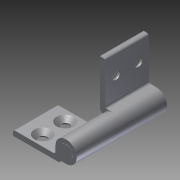
# Autodesk Inventor part: MayTec 1.62.842032085_Alu hinges, heavy, type 20 PG 40 (90)
Saved by Autodesk Inventor 2011 SP1 (Build 150282100, 282)
## iProperties
Created: 2012-12-11
Part Number: MayTec 1.62.842032085_Alu hinges, heavy, type 20 PG 40 (90)
Catalog Web Link: www.cadenas.de
Description: Alu hinges, heavy-Alu hinges, heavy
Vendor: MAYTEC
Document SubType Name: Modeling
Designer: PARTuser1
Manufacturer: MAYTEC
Density: 1 g/cm^3
Category: PARTsolutions
Company: MAYTEC
Title: MayTec 1.62.842032085_Alu hinges, heavy, type 20 PG 40 (90)
Author: Cadenas PARTsolutions
Comments: Alu hinges, heavy
PSOL_IDENT_0: {\\10.0.0.242\data_v9\23d-libs\maytec\maytec_3d\anbauzubehoer\scharniere\alu_scharniere\alu_scharnie
PSOL_IDENT_1: r_schwer.prj},278 {VTYP=3D},{NB=MayTec 1.62.842032085_Alu hinges, heavy, type 20 PG 40 (90)},{LINA=M
PSOL_IDENT_2: ayTec 1.62.842032085_Alu hinges, heavy, type 20 PG 40 (90)},{NN=Alu hinges, heavy},{DATE=14.09.2010
PSOL_IDENT_3: 08:32:09},{GEOMDATE=27.07.2010 11:58:00},{VERSION=},{LINEID=250},{LINESUBID=-1},{WBVAR=WINKEL}  {NB=
PSOL_IDENT_4: MayTec 1.62.842032085_Alu hinges, heavy, type 20 PG 40 (90)},{LINA=MayTec 1.62.842032085_Alu hinges,
PSOL_IDENT_5: heavy, type 20 PG 40 (90)},{KT=DUMMY},{PARTNR=1.62.842032085},{DESCRIPTION=Alu-Scharnier-Schwer Typ
PSOL_IDENT_6: 20 PG 40},{TYP=20.0},{AUSFHRUNG=Stahl},{H=128.75},{A=32.0},{T=20.0},{T2=86.00},{VAR=1.0},{XTRANS=Al
PSOL_IDENT_7: u hinges, heavy, type 20 PG 40},{B=100},{WINKEL=90}
CNS_NT: Alu hinges, heavy
CNS_NB: MayTec 1.62.842032085_Alu hinges, heavy, type 20 PG 40 (90)
CNS_NBSYN: MayTec $PARTNR._$XTRANS. ($WINKEL.)
CNS_LINA: MayTec 1.62.842032085_Alu hinges, heavy, type 20 PG 40 (90)
CNS_PARTNR: 1.62.842032085
CNS_DESCRIPTION: Alu hinges, heavy, type 20 PG 40
CNS_TYP: 20.0
CNS_AUSFHRUNG: Steel
CNS_H: 128.75
CNS_A: 32.0
CNS_T: 20.0
CNS_T2: 86.00
CNS_VAR: 1.0
CNS_XTRANS: Alu hinges, heavy, type 20 PG 40
CNS_B: 100
CNS_WINKEL: 90
SUPPLIER: MAYTEC
ARTICLENO: MayTec 1.62.842032085_Alu hinges, heavy, type 20 PG 40 (90)
BOMINFO: MayTec 1.62.842032085_Alu hinges, heavy, type 20 PG 40 (90)
CREATOR: CADENAS GmbH
Autodesk Inventor part; units mm, degrees
sketch "Skizze_34" plane through (0, 0, 0) normal (0, 1, 0) x (1, 0, 0)
  circle A0 centre (0, 12) radius 10
  constraints: 1 centre point
extrude "Extrusion1" add sketch "Skizze_34" along normal mid plane 2.5
sketch "Skizze_35" plane through (0, 0, 0) normal (0, 1, 0) x (1, 0, 0)
  circle A0 centre (0, 12) radius 6
  constraints: 1 centre point
extrude "Extrusion2" add sketch "Skizze_35" along normal mid plane 85.5
sketch "Skizze_36" plane through (0, -1.3, 0) normal (0, 1, 0) x (1, 0, 0)
  line L0 (-50, 24) -> (-50, 21)
  arc A0 (-50, 21) -> (-48, 19) centre (-48, 21) ccw
  line L1 (-48, 19) -> (-12, 19)
  arc A1 (-10, 17) -> (-12, 19) centre (-12, 17) ccw
  line L2 (-10, 17) -> (-10, 12)
  arc A2 (-10, 12) -> (0, 22) centre (0, 12) ccw
  line L3 (0, 22) -> (-4, 22)
  arc A3 (-5.8856, 23.3333) -> (-4, 22) centre (-4, 24) ccw
  arc A4 (-5.8856, 23.3333) -> (-6.8284, 24) centre (-6.8284, 23) ccw
  line L4 (-6.8284, 24) -> (-50, 24)
  circle A5 centre (0, 12) radius 6
  constraints: 10 end point, 10 point on circle, 6 centre point
extrude "Extrusion3" add sketch "Skizze_36" against normal blind 41.25
sketch "Skizze_37" plane through (0, 1.3, 0) normal (0, 1, 0) x (1, 0, 0)
  line L0 (-12, -38) -> (-9, -38)
  arc A0 (-9, -38) -> (-7, -36) centre (-9, -36) ccw
  line L1 (-7, -36) -> (-7, 0)
  arc A1 (-5, 2) -> (-7, 0) centre (-5, 0) ccw
  line L2 (-5, 2) -> (0, 2)
  arc A2 (0, 2) -> (-10, 12) centre (0, 12) ccw
  line L3 (-10, 12) -> (-10, 8)
  arc A3 (-11.3333, 6.1144) -> (-10, 8) centre (-12, 8) ccw
  arc A4 (-11.3333, 6.1144) -> (-12, 5.1716) centre (-11, 5.1716) ccw
  line L4 (-12, 5.1716) -> (-12, -38)
  circle A5 centre (0, 12) radius 6
  constraints: 10 end point, 10 point on circle, 6 centre point
extrude "Extrusion4" add sketch "Skizze_37" along normal blind 41.25
sketch "Sketch5" plane through (-12, 1.3, -5.1716) normal (-1, 0, 0) x (0, 0, 1)
  point P0 (25.1716, 10.13)
hole "Drilling 1" at (-12, 11.43, 20) direction (1, 0, 0) diameter 8 depth 5 countersink diameter 16 countersink angle 90
sketch "Sketch6" plane through (-12, 1.3, -5.1716) normal (-1, 0, 0) x (0, 0, 1)
  point P0 (25.1716, 31.13)
hole "Drilling 2" at (-12, 32.43, 20) direction (1, 0, 0) diameter 8 depth 5 countersink diameter 16 countersink angle 90
sketch "Sketch7" plane through (-48, -1.3, -19) normal (0, 0, 1) x (1, 0, 0)
  point P0 (16, -10.13)
hole "Drilling 3" at (-32, -11.43, -19) direction (0, 0, -1) diameter 8 depth 5 countersink diameter 16 countersink angle 90
sketch "Sketch8" plane through (-48, -1.3, -19) normal (0, 0, 1) x (1, 0, 0)
  point P0 (16, -31.13)
hole "Drilling 4" at (-32, -32.43, -19) direction (0, 0, -1) diameter 8 depth 5 countersink diameter 16 countersink angle 90
ref_plane "side_2a_XY" through (-32, -21.925, -19) normal (0, 0, 1) x (1, 0, 0)
ref_plane "side_2a_YZ" through (-32, -21.925, -19) normal (1, 0, 0) x (0, 1, 0)
ref_plane "side_2a_ZX" through (-32, -21.925, -19) normal (0, 1, 0) x (0, 0, 1)
ref_plane "side_2b_XY" through (-32, -21.925, -24) normal (0, 0, -1) x (1, 0, 0)
ref_plane "side_2b_YZ" through (-32, -21.925, -24) normal (1, 0, 0) x (0, -1, 0)
ref_plane "side_2b_ZX" through (-32, -21.925, -24) normal (0, -1, 0) x (0, 0, -1)
ref_plane "side_1b_XY" through (-7, 21.925, 20) normal (1, 0, 0) x (0, 0, -1)
ref_plane "side_1b_YZ" through (-7, 21.925, 20) normal (0, 0, -1) x (0, 1, 0)
ref_plane "side_1b_ZX" through (-7, 21.925, 20) normal (0, 1, 0) x (1, 0, 0)
ref_plane "side_3b_XY" through (-7, 21.925, 20) normal (1, 0, 0) x (0, 0, -1)
ref_plane "side_3b_YZ" through (-7, 21.925, 20) normal (0, 0, -1) x (0, 1, 0)
ref_plane "side_3b_ZX" through (-7, 21.925, 20) normal (0, 1, 0) x (1, 0, 0)
ref_plane "side_1a_XY" through (-12, 21.925, 20) normal (-1, 0, 0) x (0, 0, -1)
ref_plane "side_1a_YZ" through (-12, 21.925, 20) normal (0, 0, -1) x (0, -1, 0)
ref_plane "side_1a_ZX" through (-12, 21.925, 20) normal (0, -1, 0) x (-1, 0, 0)
ref_plane "side_3a_XY" through (-12, 21.925, 20) normal (-1, 0, 0) x (0, 0, -1)
ref_plane "side_3a_YZ" through (-12, 21.925, 20) normal (0, 0, -1) x (0, -1, 0)
ref_plane "side_3a_ZX" through (-12, 21.925, 20) normal (0, -1, 0) x (-1, 0, 0)
body "Solid1"
